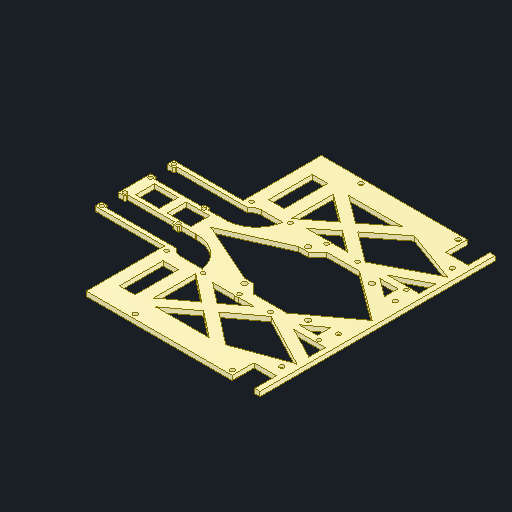
# Autodesk Inventor part: base
Saved by Autodesk Inventor 2023 (Build 270158000, 158)
## iProperties
Created: 2024-05-25
Part Number: base
Material: Nylon 6
Document SubType Name: Modeling
Designer: szymo
Density: 1.12 g/cm^3
Appearance: Nylon 6
Mass: 52.6414 g
Surface Area: 374.205 cm^2
Volume: 47.0013 cm^3
Author: szymo
Autodesk Inventor part; units mm, degrees
ref_plane "YZ Plane" through (0, 0, 0) normal (1, 0, 0) x (0, 1, 0)
ref_plane "XZ Plane" through (0, 0, 0) normal (0, 1, 0) x (-1, 0, 0)
ref_plane "XY Plane" through (0, 0, 0) normal (0, 0, 1) x (1, 0, 0)
sketch "Sketch1" plane through (0, 0, 0) normal (0, 1, 0) x (-1, 0, 0)
  line L0 (99, 89) -> (-99, 89)
  line L1 (-99, 89) -> (-99, -89)
  line L2 (-99, -89) -> (99, -89)
  line L3 (99, -89) -> (99, 89)
  line L4 (99, 89) -> (-99, -89) construction
  line L5 (-99, 89) -> (99, -89) construction
  line L6 (-85, 89) -> (-85, -89)
  line L7 (-64, 89) -> (-64, 72.5)
  line L8 (-64, 72.5) -> (-81, 72.5)
  line L9 (-81, -72.5) -> (-64, -72.5)
  line L10 (-64, -72.5) -> (-64, -89)
  line L11 (-81, -89) -> (-81, 89)
  point P0 (0, 0)
  dimension "d0" = 198
  dimension "d1" = 178
  dimension "d2" = 14
  dimension "d3" = 16.5
  dimension "d4" = 16.5
  dimension "d9" = 4
  dimension "d10" = 17
  dimension "d11" = 17
  constraints: 24 end point, 8 point on line, 6 perpendicular, 2 horizontal, 2 midpoint, 2 parallel, 1 vertical
  measures "d0" distance of L2.end L1.end
  measures "d1" distance of L1.end L0.end
  measures "d2" distance between parallel lines of L6 L1
  measures "d3" distance between parallel lines of L0 L8
  measures "d4" distance between parallel lines of L9 L2
  measures "d9" distance between parallel lines of L11 L6
  measures "d10" distance between parallel lines of L10 L11
  measures "d11" distance between parallel lines of L11 L7
extrude "Extrusion1" add sketch "Sketch1" along normal blind 3.5 contours L3 L2 L10 L9 L11 L8 L7 L0 | L11 L2 L6 L0
sketch "Sketch2" plane through (0, 0, 0) normal (0, -1, 0) x (1, 0, 0)
  circle A0 centre (77, -64.5) radius 1.2295
  circle A1 centre (77, -21.5) radius 1.2295
  circle A2 centre (77, 21.5) radius 1.2295
  circle A3 centre (77, 64.5) radius 1.2295
  line L0 (79, 89) -> (79, 88)
  line L1 (-46.5, 89) -> (79, 89)
  line L2 (-46.5, 89) -> (-46.5, 73)
  line L3 (-39.246, 73) -> (-46.5, 73)
  spline S0 degree 3 poles (-38.725, 73.0306) (-38.9029, 73.01) (-39.0786, 73) (-39.246, 73) knots 0 0 0 0 1 1 1 1
  line L4 (-38.725, 88) -> (-38.725, 73.0306)
  line L5 (-24.275, 73.0306) -> (-24.275, 88)
  line L6 (-16.5, 73) -> (-23.754, 73)
  arc A4 (-9.5, 82) -> (-16.5, 73) centre (-6.5148, 72.456) ccw
  arc A5 (-1.5, 86) -> (-9.5, 82) centre (-1.5, 76) ccw
  circle A6 centre (70, 79.5) radius 1.75
  circle A7 centre (-13, 85.5) radius 2.3
  circle A8 centre (60.5017, 85.4375) radius 2.3
  circle A9 centre (70, -82.5) radius 1.75
  arc A10 (58.4256, -82) -> (56.6186, -83.1429) centre (58.4256, -84) ccw
  arc A11 (52.101, -86) -> (56.6186, -83.1429) centre (52.101, -81) ccw
  arc A12 (-9.5, -82) -> (-1.5, -86) centre (-1.5, -76) ccw
  arc A13 (-16.5, -73) -> (-9.5, -82) centre (-6.5148, -72.456) ccw
  line L7 (-16.5, -73) -> (-23.754, -73)
  spline S1 degree 3 poles (-23.754, -73) (-23.9214, -73) (-24.0971, -73.01) (-24.275, -73.0306) knots 0 0 0 0 1 1 1 1
  line L8 (-24.275, -73.0306) -> (-24.275, -88)
  line L9 (-24.275, -88) -> (-38.725, -88)
  line L10 (-38.725, -88) -> (-38.725, -73.0306)
  spline S2 degree 3 poles (-38.725, -73.0306) (-38.9029, -73.01) (-39.0786, -73) (-39.246, -73) knots 0 0 0 0 1 1 1 1
  line L11 (-39.246, -73) -> (-46.5, -73)
  line L12 (-46.5, -89) -> (-46.5, -73)
  line L13 (-46.5, -89) -> (79, -89)
  line L14 (79, -89) -> (79, -88)
  arc A14 (68.9282, -76) -> (66.9487, -77.7143) centre (68.9282, -78) ccw
  arc A15 (62, -82) -> (66.9487, -77.7143) centre (62, -77) ccw
  line L15 (62, -82) -> (58.4256, -82)
  circle A16 centre (-13, -85.5) radius 2.3
  circle A17 centre (60.5017, -85.4375) radius 2.3
  line L16 (73, 83) -> (73, 78)
  line L17 (52.101, 86) -> (-1.5, 86)
  arc A18 (71, 76) -> (73, 78) centre (71, 78) ccw
  arc A19 (78, 88) -> (73, 83) centre (78, 83) ccw
  line L18 (79, 88) -> (78, 88)
  line L19 (-24.275, 88) -> (-38.725, 88)
  spline S3 degree 3 poles (-23.754, 73) (-23.9214, 73) (-24.0971, 73.01) (-24.275, 73.0306) knots 0 0 0 0 1 1 1 1
  arc A20 (56.6186, 83.1429) -> (52.101, 86) centre (52.101, 81) ccw
  arc A21 (56.6186, 83.1429) -> (58.4256, 82) centre (58.4256, 84) ccw
  line L20 (62, 82) -> (58.4256, 82)
  arc A22 (66.9487, 77.7143) -> (62, 82) centre (62, 77) ccw
  arc A23 (66.9487, 77.7143) -> (68.9282, 76) centre (68.9282, 78) ccw
  line L21 (71, 76) -> (68.9282, 76)
  arc A24 (73, -78) -> (71, -76) centre (71, -78) ccw
  line L22 (71, -76) -> (68.9282, -76)
  line L23 (52.101, -86) -> (-1.5, -86)
  line L24 (79, -88) -> (78, -88)
  arc A25 (73, -83) -> (78, -88) centre (78, -83) ccw
  line L25 (73, -83) -> (73, -78)
  point P0 (0, 0)
  point P1 (-13, -85.5)
  point P2 (-13, 85.5)
  constraints: 6 coincident
hole "m3" at (-13, 0, -85.5) at (60.5017, 0, -85.4375) at (-13, 0, 85.5) at (60.5017, 0, 85.4375) at (77, 0, 64.5) at (77, 0, 21.5) at (77, 0, -21.5) at (77, 0, -64.5) direction (0, 1, 0) diameter 3.6 end through all countersink diameter 6.7 countersink angle 90 clearance for "Countersunk Flat Head Screw ISO 2009/7046" size "M3" standard "ISO"
sketch "Sketch3" plane through (0, 0, 0) normal (0, -1, 0) x (1, 0, 0)
  circle A0 centre (-96.5, -27.3) radius 1.75
  circle A1 centre (-96.5, -9.7) radius 1.75
  circle A2 centre (-96.5, 9.7) radius 1.75
  circle A3 centre (-96.5, 27.3) radius 1.75
  circle A4 centre (-56, 9.7) radius 1.75
  circle A5 centre (-56, -9.7) radius 1.75
  circle A6 centre (-42.5596, -32.1689) radius 1.5
  circle A7 centre (-42.5596, 32.1689) radius 1.75
  circle A8 centre (-13.9698, 33) radius 1.75
  circle A9 centre (13.5198, 33) radius 1.75
  circle A10 centre (37.0073, 33) radius 1.75
  circle A11 centre (73.7355, 33) radius 1.75
  circle A12 centre (73.7355, -33) radius 1.75
  circle A13 centre (37.0073, -33) radius 1.75
  circle A14 centre (-96.5, -27.3) radius 1.75
  circle A15 centre (73.7355, -33) radius 1.75
  circle A16 centre (13.5198, -33) radius 1.75
  circle A17 centre (-42.5596, -32.1689) radius 1.75
  circle A18 centre (-13.9698, -33) radius 1.75
  arc A19 (-94, -25.8) -> (-95, -24.8) centre (-95, -25.8) ccw
  line L0 (-95, -24.8) -> (-99, -24.8)
  line L1 (-99, -29.8) -> (-99, -24.8)
  line L2 (-48.6566, -29.8) -> (-99, -29.8)
  arc A20 (-47.7313, -30.4207) -> (-48.6566, -29.8) centre (-48.6566, -30.8) ccw
  arc A21 (-46.5, -35.5) -> (-47.7313, -30.4207) centre (-63.78, -37) ccw
  line L3 (79, -35.5) -> (-46.5, -35.5)
  line L4 (79, -35.5) -> (79, -30.5)
  line L5 (79, -30.5) -> (-33.3917, -30.5)
  arc A22 (-40.5373, -26.8) -> (-33.3917, -30.5) centre (-33.3917, -21.75) ccw
  line L6 (-40.5373, -26.8) -> (-41.9987, -26.8)
  spline S0 degree 3 poles (-46.8237, -26.8) (-46.5789, -26.8) (-46.2862, -26.7761) (-45.5332, -26.6913) (-44.9243, -26.6) (-44.4112, -26.6) (-43.8981, -26.6) (-43.2892, -26.6913) (-42.5362, -26.7761) (-42.2435, -26.8) (-41.9987, -26.8) knots 0 0 0 0 0.161475 0.161475 0.5 0.5 0.5 0.838525 0.838525 1 1 1 1
  line L7 (-46.8237, -26.8) -> (-94, -26.8)
  line L8 (-94, -26.8) -> (-94, -25.8)
  line L9 (28.681, 30.5) -> (45.3337, 30.5)
  circle A23 centre (37.0073, 33) radius 1.75
  circle A24 centre (-96.5, 27.3) radius 1.75
  circle A25 centre (73.7355, 33) radius 1.75
  circle A26 centre (13.5198, 33) radius 1.75
  circle A27 centre (-42.5596, 32.1689) radius 1.75
  circle A28 centre (-13.9698, 33) radius 1.75
  arc A29 (-95, 24.8) -> (-94, 25.8) centre (-95, 25.8) ccw
  line L10 (-94, 26.8) -> (-94, 25.8)
  line L11 (-46.8237, 26.8) -> (-94, 26.8)
  spline S1 degree 3 poles (-46.8237, 26.8) (-46.5789, 26.8) (-46.2862, 26.7761) (-45.5332, 26.6913) (-44.9243, 26.6) (-44.4112, 26.6) (-43.8981, 26.6) (-43.2892, 26.6913) (-42.5362, 26.7761) (-42.2435, 26.8) (-41.9987, 26.8) knots 0 0 0 0 0.161475 0.161475 0.5 0.5 0.5 0.838525 0.838525 1 1 1 1
  line L12 (-40.5373, 26.8) -> (-41.9987, 26.8)
  arc A30 (-33.3917, 30.5) -> (-40.5373, 26.8) centre (-33.3917, 21.75) ccw
  line L13 (79, 30.5) -> (-33.3917, 30.5)
  line L14 (79, 35.5) -> (79, 30.5)
  line L15 (79, 35.5) -> (-46.5, 35.5)
  arc A31 (-47.7313, 30.4207) -> (-46.5, 35.5) centre (-63.78, 37) ccw
  arc A32 (-48.6566, 29.8) -> (-47.7313, 30.4207) centre (-48.6566, 30.8) ccw
  line L16 (-48.6566, 29.8) -> (-99, 29.8)
  line L17 (-99, 29.8) -> (-99, 24.8)
  line L18 (-95, 24.8) -> (-99, 24.8)
  point P0 (0, 0)
  constraints: 16 coincident
hole "m2.5" at (73.7355, 0, -33) at (37.0073, 0, -33) at (13.5198, 0, -33) at (-13.9698, 0, -33) at (-42.5596, 0, -32.1689) at (73.7355, 0, 33) at (37.0073, 0, 33) at (13.5198, 0, 33) at (-13.9698, 0, 33) at (-42.5596, 0, 32.1689) at (-56, 0, 9.7) at (-56, 0, -9.7) at (-96.5, 0, -9.7) at (-96.5, 0, 9.7) at (-96.5, 0, 27.3) at (-96.5, 0, -27.3) direction (0, 1, 0) diameter 3.1 end through all countersink diameter 5.8 countersink angle 90 clearance for "Countersunk Flat Head Screw ISO 2009/7046" size "M2.5" standard "ISO"
sketch "Sketch6" plane through (0, 0, 0) normal (0, -1, 0) x (1, 0, 0)
  line L0 (60, 27.5) -> (5, 27.5) projected
  line L1 (5, 27.5) -> (5, -27.5) projected
  line L2 (5, -27.5) -> (60, -27.5) projected
  line L3 (60, -27.5) -> (60, 27.5) projected
  circle A0 centre (48.73, 26.5) radius 0.325 projected
  circle A1 centre (45, 26.5) radius 0.325 projected
  circle A2 centre (46.27, 26.5) radius 0.325 projected
  circle A3 centre (52.54, 26.5) radius 0.325 projected
  circle A4 centre (56.6, 24.1) radius 1.6 projected
  circle A5 centre (50, 26.5) radius 0.325 projected
  circle A6 centre (51.27, 26.5) radius 0.325 projected
  circle A7 centre (42.46, 26.5) radius 0.325 projected
  circle A8 centre (43.73, 26.5) radius 0.325 projected
  circle A9 centre (8.4, 24.1) radius 1.6 projected
  circle A10 centre (7, 15) radius 0.35 projected
  circle A11 centre (9.5, 15) radius 0.35 projected
  circle A12 centre (9.5, 7.75) radius 0.35 projected
  circle A13 centre (7, 7.75) radius 0.35 projected
  circle A14 centre (9.5, 0.5) radius 0.35 projected
  circle A15 centre (56.6, -24.1) radius 1.6 projected
  circle A16 centre (51.27, -26.5) radius 0.325 projected
  circle A17 centre (52.54, -26.5) radius 0.325 projected
  circle A18 centre (48.73, -26.5) radius 0.325 projected
  circle A19 centre (50, -26.5) radius 0.325 projected
  circle A20 centre (45, -26.5) radius 0.325 projected
  circle A21 centre (46.27, -26.5) radius 0.325 projected
  circle A22 centre (9.5, -6.75) radius 0.35 projected
  circle A23 centre (9.5, -14) radius 0.35 projected
  circle A24 centre (7, 0.5) radius 0.35 projected
  circle A25 centre (7, -6.75) radius 0.35 projected
  circle A26 centre (42.46, -26.5) radius 0.325 projected
  circle A27 centre (43.73, -26.5) radius 0.325 projected
  circle A28 centre (7, -14) radius 0.35 projected
  circle A29 centre (8.4, -24.1) radius 1.6 projected
  point P0 (0, 0)
  constraints: 4 coincident
hole "insert_stack" at (8.4, 0, -24.1) at (8.4, 0, 24.1) at (56.6, 0, 24.1) at (56.6, 0, -24.1) direction (0, 1, 0) diameter 4 depth 4.5 counterbore diameter 4.6 counterbore depth 1
sketch "Sketch5" plane through (0, 0, 0) normal (0, 1, 0) x (1, 0, 0)
  line L0 (-36.8852, -40.5) -> (-31.5, -40.5)
  line L1 (-31.5, -40.5) -> (-26.1148, -40.5)
  line L2 (-26.1148, -40.5) -> (-26.1148, -68.2)
  line L3 (-26.1148, -68.2) -> (-36.8852, -68.2)
  line L4 (-36.8852, -68.2) -> (-36.8852, -40.5)
  line L5 (-26.1148, 40.5) -> (-31.5, 40.5)
  line L6 (-31.5, 40.5) -> (-36.8852, 40.5)
  line L7 (-36.8852, 40.5) -> (-36.8852, 68.2)
  line L8 (-36.8852, 68.2) -> (-26.1148, 68.2)
  line L9 (-26.1148, 68.2) -> (-26.1148, 40.5)
  arc A0 (-99, -28.7697) -> (-99, -25.8303) centre (-96.5, -27.3) ccw
  line L10 (-99, -11.1697) -> (-99, -25.8303)
  arc A1 (-99, -11.1697) -> (-99, -8.2303) centre (-96.5, -9.7) ccw
  line L11 (-99, 8.2303) -> (-99, -8.2303)
  arc A2 (-99, 8.2303) -> (-99, 11.1697) centre (-96.5, 9.7) ccw
  line L12 (-99, 25.8303) -> (-99, 11.1697)
  arc A3 (-99, 25.8303) -> (-99, 28.7697) centre (-96.5, 27.3) ccw
  line L13 (-99, 89) -> (-99, 28.7697)
  line L14 (64, 89) -> (-99, 89)
  line L15 (64, 72.5) -> (64, 89)
  line L16 (81, 72.5) -> (64, 72.5)
  line L17 (81, 89) -> (81, 72.5)
  line L18 (85, 89) -> (81, 89)
  line L19 (85, -89) -> (85, 89)
  line L20 (81, -89) -> (85, -89)
  line L21 (81, -72.5) -> (81, -89)
  line L22 (64, -72.5) -> (81, -72.5)
  line L23 (64, -89) -> (64, -72.5)
  line L24 (-99, -89) -> (64, -89)
  line L25 (-99, -28.7697) -> (-99, -89)
  circle A4 centre (77, 64.5) radius 3.35
  circle A5 centre (77, -21.5) radius 3.35
  circle A6 centre (60.5017, -85.4375) radius 3.35
  circle A7 centre (60.5017, 85.4375) radius 3.35
  circle A8 centre (-13, 85.5) radius 3.35
  circle A9 centre (-13, -85.5) radius 3.35
  circle A10 centre (77, -64.5) radius 3.35
  circle A11 centre (77, 21.5) radius 3.35
  circle A12 centre (-56, 9.7) radius 2.9
  circle A13 centre (-42.5596, -32.1689) radius 2.9
  circle A14 centre (13.5198, -33) radius 2.9
  circle A15 centre (73.7355, -33) radius 2.9
  circle A16 centre (-13.9698, 33) radius 2.9
  circle A17 centre (37.0073, 33) radius 2.9
  circle A18 centre (73.7355, 33) radius 2.9
  circle A19 centre (13.5198, 33) radius 2.9
  circle A20 centre (-42.5596, 32.1689) radius 2.9
  circle A21 centre (37.0073, -33) radius 2.9
  circle A22 centre (-13.9698, -33) radius 2.9
  circle A23 centre (-56, -9.7) radius 2.9
  arc A24 (56.6186, 83.1429) -> (58.4256, 82) centre (58.4256, 84) ccw
  arc A25 (56.6186, 83.1429) -> (52.101, 86) centre (52.101, 81) ccw
  line L26 (52.101, 86) -> (-1.5, 86)
  arc A26 (-1.5, 86) -> (-9.5, 82) centre (-1.5, 76) ccw
  arc A27 (-9.5, 82) -> (-16.5, 73) centre (-6.5148, 72.456) ccw
  line L27 (-16.5, 73) -> (-23.754, 73)
  spline S0 degree 3 poles (-23.754, 73) (-23.9214, 73) (-24.0971, 73.01) (-24.275, 73.0306) knots 0 0 0 0 1 1 1 1
  line L28 (-24.275, 73.0306) -> (-24.275, 88)
  line L29 (-24.275, 88) -> (-38.725, 88)
  line L30 (-38.725, 88) -> (-38.725, 73.0306)
  spline S1 degree 3 poles (-38.725, 73.0306) (-38.9029, 73.01) (-39.0786, 73) (-39.246, 73) knots 0 0 0 0 1 1 1 1
  line L31 (-39.246, 73) -> (-46.5, 73)
  line L32 (-46.5, 89) -> (-46.5, 73)
  line L33 (-46.5, 89) -> (79, 89)
  line L34 (79, 89) -> (79, 86)
  arc A28 (79, 86) -> (74.3229, 81.0104) centre (79.3229, 81.0104) ccw
  line L35 (74.3229, 81.0104) -> (74.3229, 78)
  arc A29 (72.3229, 76) -> (74.3229, 78) centre (72.3229, 78) ccw
  line L36 (72.3229, 76) -> (68.9282, 76)
  arc A30 (66.9487, 77.7143) -> (68.9282, 76) centre (68.9282, 78) ccw
  arc A31 (66.9487, 77.7143) -> (62, 82) centre (62, 77) ccw
  line L37 (62, 82) -> (58.4256, 82)
  arc A32 (-95, 24.8) -> (-94, 25.8) centre (-95, 25.8) ccw
  line L38 (-95, 24.8) -> (-99, 24.8)
  line L39 (-99, 29.8) -> (-99, 24.8)
  line L40 (-48.6566, 29.8) -> (-99, 29.8)
  arc A33 (-48.6566, 29.8) -> (-47.7313, 30.4207) centre (-48.6566, 30.8) ccw
  arc A34 (-47.7313, 30.4207) -> (-46.5, 35.5) centre (-63.78, 37) ccw
  line L41 (79, 35.5) -> (-46.5, 35.5)
  line L42 (79, 35.5) -> (79, 30.5)
  line L43 (79, 30.5) -> (-33.3917, 30.5)
  arc A35 (-33.3917, 30.5) -> (-40.5373, 26.8) centre (-33.3917, 21.75) ccw
  line L44 (-40.5373, 26.8) -> (-41.9987, 26.8)
  spline S2 degree 3 poles (-46.8237, 26.8) (-46.5789, 26.8) (-46.2862, 26.7761) (-45.5332, 26.6913) (-44.9243, 26.6) (-44.4112, 26.6) (-43.8981, 26.6) (-43.2892, 26.6913) (-42.5362, 26.7761) (-42.2435, 26.8) (-41.9987, 26.8) knots 0 0 0 0 0.161475 0.161475 0.5 0.5 0.5 0.838525 0.838525 1 1 1 1
  line L45 (-46.8237, 26.8) -> (-94, 26.8)
  line L46 (-94, 26.8) -> (-94, 25.8)
  arc A36 (-57.5, 12.2) -> (-58.5, 11.2) centre (-57.5, 11.2) ccw
  line L47 (-57.5, 12.2) -> (-54.5, 12.2)
  arc A37 (-53.5, 11.2) -> (-54.5, 12.2) centre (-54.5, 11.2) ccw
  line L48 (-53.5, 11.2) -> (-53.5, 10.2)
  line L49 (-53.5, 10.2) -> (-46.8237, 10.2)
  spline S3 degree 3 poles (-41.9987, 10.2) (-42.2435, 10.2) (-42.5362, 10.2239) (-43.2892, 10.3087) (-43.8981, 10.4) (-44.4112, 10.4) (-44.9243, 10.4) (-45.5332, 10.3087) (-46.2862, 10.2239) (-46.5789, 10.2) (-46.8237, 10.2) knots 0 0 0 0 0.161475 0.161475 0.5 0.5 0.5 0.838525 0.838525 1 1 1 1
  line L50 (-41.9987, 10.2) -> (-41.148, 10.2)
  line L51 (-41.148, 10.2) -> (-41.148, 7.2)
  line L52 (-41.148, 7.2) -> (-99, 7.2)
  line L53 (-99, 7.2) -> (-99, 12.2)
  line L54 (-99, 12.2) -> (-95, 12.2)
  arc A38 (-94, 11.2) -> (-95, 12.2) centre (-95, 11.2) ccw
  line L55 (-94, 10.2) -> (-94, 11.2)
  line L56 (-94, 10.2) -> (-58.5, 10.2)
  line L57 (-58.5, 10.2) -> (-58.5, 11.2)
  arc A39 (-58.5, -11.2) -> (-57.5, -12.2) centre (-57.5, -11.2) ccw
  line L58 (-58.5, -10.2) -> (-58.5, -11.2)
  line L59 (-94, -10.2) -> (-58.5, -10.2)
  line L60 (-94, -10.2) -> (-94, -11.2)
  arc A40 (-95, -12.2) -> (-94, -11.2) centre (-95, -11.2) ccw
  line L61 (-99, -12.2) -> (-95, -12.2)
  line L62 (-99, -7.2) -> (-99, -12.2)
  line L63 (-41.148, -7.2) -> (-99, -7.2)
  line L64 (-41.148, -10.2) -> (-41.148, -7.2)
  line L65 (-41.9987, -10.2) -> (-41.148, -10.2)
  spline S4 degree 3 poles (-41.9987, -10.2) (-42.2435, -10.2) (-42.5362, -10.2239) (-43.2892, -10.3087) (-43.8981, -10.4) (-44.4112, -10.4) (-44.9243, -10.4) (-45.5332, -10.3087) (-46.2862, -10.2239) (-46.5789, -10.2) (-46.8237, -10.2) knots 0 0 0 0 0.161475 0.161475 0.5 0.5 0.5 0.838525 0.838525 1 1 1 1
  line L66 (-53.5, -10.2) -> (-46.8237, -10.2)
  line L67 (-53.5, -11.2) -> (-53.5, -10.2)
  arc A41 (-54.5, -12.2) -> (-53.5, -11.2) centre (-54.5, -11.2) ccw
  line L68 (-57.5, -12.2) -> (-54.5, -12.2)
  arc A42 (-94, -25.8) -> (-95, -24.8) centre (-95, -25.8) ccw
  line L69 (-94, -26.8) -> (-94, -25.8)
  line L70 (-46.8237, -26.8) -> (-94, -26.8)
  spline S5 degree 3 poles (-46.8237, -26.8) (-46.5789, -26.8) (-46.2862, -26.7761) (-45.5332, -26.6913) (-44.9243, -26.6) (-44.4112, -26.6) (-43.8981, -26.6) (-43.2892, -26.6913) (-42.5362, -26.7761) (-42.2435, -26.8) (-41.9987, -26.8) knots 0 0 0 0 0.161475 0.161475 0.5 0.5 0.5 0.838525 0.838525 1 1 1 1
  line L71 (-40.5373, -26.8) -> (-41.9987, -26.8)
  arc A43 (-40.5373, -26.8) -> (-33.3917, -30.5) centre (-33.3917, -21.75) ccw
  line L72 (79, -30.5) -> (-33.3917, -30.5)
  line L73 (79, -35.5) -> (79, -30.5)
  line L74 (79, -35.5) -> (-46.5, -35.5)
  arc A44 (-46.5, -35.5) -> (-47.7313, -30.4207) centre (-63.78, -37) ccw
  arc A45 (-47.7313, -30.4207) -> (-48.6566, -29.8) centre (-48.6566, -30.8) ccw
  line L75 (-48.6566, -29.8) -> (-99, -29.8)
  line L76 (-99, -29.8) -> (-99, -24.8)
  line L77 (-95, -24.8) -> (-99, -24.8)
  arc A46 (58.4256, -82) -> (56.6186, -83.1429) centre (58.4256, -84) ccw
  line L78 (62, -82) -> (58.4256, -82)
  arc A47 (62, -82) -> (66.9487, -77.7143) centre (62, -77) ccw
  arc A48 (68.9282, -76) -> (66.9487, -77.7143) centre (68.9282, -78) ccw
  line L79 (72.3229, -76) -> (68.9282, -76)
  arc A49 (74.3229, -78) -> (72.3229, -76) centre (72.3229, -78) ccw
  line L80 (74.3229, -81.0104) -> (74.3229, -78)
  arc A50 (74.3229, -81.0104) -> (79, -86) centre (79.3229, -81.0104) ccw
  line L81 (79, -89) -> (79, -86)
  line L82 (-46.5, -89) -> (79, -89)
  line L83 (-46.5, -89) -> (-46.5, -73)
  line L84 (-39.246, -73) -> (-46.5, -73)
  spline S6 degree 3 poles (-38.725, -73.0306) (-38.9029, -73.01) (-39.0786, -73) (-39.246, -73) knots 0 0 0 0 1 1 1 1
  line L85 (-38.725, -88) -> (-38.725, -73.0306)
  line L86 (-24.275, -88) -> (-38.725, -88)
  line L87 (-24.275, -73.0306) -> (-24.275, -88)
  spline S7 degree 3 poles (-23.754, -73) (-23.9214, -73) (-24.0971, -73.01) (-24.275, -73.0306) knots 0 0 0 0 1 1 1 1
  line L88 (-16.5, -73) -> (-23.754, -73)
  arc A51 (-16.5, -73) -> (-9.5, -82) centre (-6.5148, -72.456) ccw
  arc A52 (-9.5, -82) -> (-1.5, -86) centre (-1.5, -76) ccw
  line L89 (52.101, -86) -> (-1.5, -86)
  arc A53 (52.101, -86) -> (56.6186, -83.1429) centre (52.101, -81) ccw
  line L90 (85, 89) -> (99, 89)
  line L91 (99, 89) -> (99, -89)
  line L92 (85, -89) -> (99, -89)
  line L93 (85, 89) -> (85, -89)
  line L94 (70, 72) -> (79, 72)
  arc A54 (79, 72) -> (81, 74) centre (79, 74) ccw
  line L95 (81, 74) -> (81, 89)
  line L96 (81, 89) -> (85, 89)
  line L97 (85, 89) -> (85, -89)
  line L98 (81, -89) -> (85, -89)
  line L99 (81, -89) -> (81, -74)
  arc A55 (81, -74) -> (79, -72) centre (79, -74) ccw
  line L100 (79, -72) -> (70, -72)
  line L101 (70, -57) -> (70, -72)
  line L102 (70, -57) -> (79, -57)
  arc A56 (79, -57) -> (81, -55) centre (79, -55) ccw
  line L103 (81, -55) -> (81, -31)
  arc A57 (81, -31) -> (79, -29) centre (79, -31) ccw
  line L104 (79, -29) -> (70, -29)
  line L105 (70, -14) -> (70, -29)
  line L106 (70, -14) -> (79, -14)
  arc A58 (79, -14) -> (81, -12) centre (79, -12) ccw
  line L107 (81, -12) -> (81, 12)
  arc A59 (81, 12) -> (79, 14) centre (79, 12) ccw
  line L108 (79, 14) -> (70, 14)
  line L109 (70, 29) -> (70, 14)
  line L110 (70, 29) -> (79, 29)
  arc A60 (79, 29) -> (81, 31) centre (79, 31) ccw
  line L111 (81, 31) -> (81, 55)
  arc A61 (81, 55) -> (79, 57) centre (79, 55) ccw
  line L112 (79, 57) -> (70, 57)
  line L113 (70, 72) -> (70, 57)
  line L114 (60, -27.5) -> (5, -27.5)
  line L115 (5, -27.5) -> (5, 27.5)
  line L116 (5, 27.5) -> (60, 27.5)
  line L117 (60, 27.5) -> (60, -27.5)
  circle A62 centre (56.6, -24.1) radius 1.6
  circle A63 centre (8.4, -24.1) radius 1.6
  circle A64 centre (56.6, 24.1) radius 1.6
  circle A65 centre (8.4, 24.1) radius 1.6
  line L118 (-37.3852, 68.7) -> (-37.3852, 40)
  line L119 (-37.3852, 40) -> (-31.5, 40)
  line L120 (-31.5, 40) -> (-25.6148, 40)
  line L121 (-25.6148, 40) -> (-25.6148, 68.7)
  line L122 (-25.6148, 68.7) -> (-37.3852, 68.7)
  line L123 (-37.3852, -40) -> (-31.5, -40)
  line L124 (-31.5, -40) -> (-25.6148, -40)
  line L125 (-25.6148, -40) -> (-25.6148, -68.7)
  line L126 (-25.6148, -68.7) -> (-37.3852, -68.7)
  line L127 (-37.3852, -68.7) -> (-37.3852, -40)
  line L128 (81, 55) -> (81, 57)
  line L129 (81, 57) -> (79, 57)
  line L130 (-46.5, -73) -> (64, -73)
  line L131 (-46.5, 73) -> (64, 73)
  line L132 (81, 57) -> (37.0404, 73)
  line L133 (79, -57) -> (81, -57)
  line L134 (81, -57) -> (81, -55)
  line L135 (81, -57) -> (37.0404, -73)
  line L136 (-46.5, 73) -> (-46.5, 35.5)
  line L137 (-37.3852, 73) -> (-37.3852, 68.7)
  line L138 (-37.3852, 40) -> (-37.3852, 35.5)
  line L139 (-25.6148, 40) -> (-25.6148, 35.5)
  line L140 (-25.6148, 68.7) -> (-25.6148, 73)
  line L141 (-16.5, 73) -> (-16.5, 35.5)
  line L142 (-46.5, -35.5) -> (-46.5, -73)
  line L143 (-37.3852, -35.5) -> (-37.3852, -40)
  line L144 (-37.3852, -68.7) -> (-37.3852, -73)
  line L145 (-25.6148, -68.7) -> (-25.6148, -73)
  line L146 (-25.6148, -40) -> (-25.6148, -35.5)
  line L147 (-16.5, -73) -> (-16.5, -35.5)
  line L148 (79, 35.5) -> (81, 35.5)
  line L149 (79, 30.5) -> (80.9365, 30.5)
  line L150 (79, -35.5) -> (81, -35.5)
  line L151 (79, -30.5) -> (80.9365, -30.5)
  line L152 (53.1, 27.6) -> (60.1, 27.6)
  line L153 (60.1, 27.6) -> (60.1, 20.6)
  line L154 (60.1, 20.6) -> (53.1, 20.6)
  line L155 (53.1, 20.6) -> (53.1, 27.6)
  line L156 (53.1, 27.6) -> (60.1, 20.6) construction
  line L157 (60.1, 27.6) -> (53.1, 20.6) construction
  line L158 (53.1, -20.6) -> (60.1, -20.6)
  line L159 (60.1, -20.6) -> (60.1, -27.6)
  line L160 (60.1, -27.6) -> (53.1, -27.6)
  line L161 (53.1, -27.6) -> (53.1, -20.6)
  line L162 (53.1, -20.6) -> (60.1, -27.6) construction
  line L163 (60.1, -20.6) -> (53.1, -27.6) construction
  line L164 (4.9, 27.6) -> (11.9, 27.6)
  line L165 (11.9, 27.6) -> (11.9, 20.6)
  line L166 (11.9, 20.6) -> (4.9, 20.6)
  line L167 (4.9, 20.6) -> (4.9, 27.6)
  line L168 (4.9, 27.6) -> (11.9, 20.6) construction
  line L169 (11.9, 27.6) -> (4.9, 20.6) construction
  line L170 (4.9, -27.6) -> (11.9, -27.6)
  line L171 (11.9, -27.6) -> (11.9, -20.6)
  line L172 (11.9, -20.6) -> (4.9, -20.6)
  line L173 (4.9, -20.6) -> (4.9, -27.6)
  line L174 (4.9, -27.6) -> (11.9, -20.6) construction
  line L175 (11.9, -27.6) -> (4.9, -20.6) construction
  line L176 (81, 57) -> (39.6917, 35.5)
  line L177 (81, -57) -> (39.6917, -35.5)
  line L178 (81, 0) -> (39.6917, 30.5)
  line L179 (81, 0) -> (39.6917, -30.5)
  line L180 (39.6917, 35.5) -> (39.6917, 30.5)
  line L181 (39.6917, -30.5) -> (39.6917, -35.5)
  line L182 (11.9, 20.6) -> (21.8, 30.5)
  line L183 (11.9, -20.6) -> (21.8, -30.5)
  line L184 (4.9, 20.6) -> (-5, 30.5)
  line L185 (4.9, -20.6) -> (-5, -30.5)
  line L186 (37.0404, 73) -> (-13.9698, 33) construction
  line L187 (37.0404, -73) -> (-13.9698, -33) construction
  line L188 (-16.5, 73) -> (37.0073, 33) construction
  line L189 (-16.5, -73) -> (37.0073, -33) construction
  line L190 (-16.5, 68.0058) -> (26.9825, 35.5)
  line L191 (-9.8194, 73) -> (40.3437, 35.5)
  line L192 (-16.5, 36.0991) -> (30.558, 73)
  line L193 (43.5227, 73) -> (-4.2994, 35.5)
  line L194 (30.558, -73) -> (-16.5, -36.0991)
  line L195 (-16.5, -68.0058) -> (26.9825, -35.5)
  line L196 (40.3437, -35.5) -> (-9.8194, -73)
  line L197 (-4.2994, -35.5) -> (43.5227, -73)
  line L198 (-46.8237, 26.8) -> (-41.9987, 26.8)
  line L199 (-41.9987, 10.2) -> (-46.8237, 10.2)
  line L200 (-46.8237, -10.2) -> (-41.9987, -10.2)
  line L201 (-41.9987, -26.8) -> (-46.8237, -26.8)
  line L202 (-46.5, 35.5) -> (-46.5, 29.8)
  line L203 (-46.5, 29.8) -> (-48.6566, 29.8)
  line L204 (-48.6566, -29.8) -> (-46.5, -29.8)
  line L205 (-46.5, -29.8) -> (-46.5, -35.5)
  line L206 (-99, 7.2) -> (-91, 7.2)
  line L207 (-91, 7.2) -> (-91, -7.2)
  line L208 (-91, -7.2) -> (-99, -7.2)
  line L209 (-99, -7.2) -> (-99, 7.2)
  line L210 (-41.148, 7.2) -> (-49.148, 7.2)
  line L211 (-49.148, 7.2) -> (-49.148, -7.2)
  line L212 (-49.148, -7.2) -> (-41.148, -7.2)
  line L213 (-41.148, -7.2) -> (-41.148, 7.2)
  line L214 (-73.074, 7.2) -> (-67.074, 7.2)
  line L215 (-67.074, 7.2) -> (-67.074, -7.2)
  line L216 (-67.074, -7.2) -> (-73.074, -7.2)
  line L217 (-73.074, -7.2) -> (-73.074, 7.2)
  circle A66 centre (-41.148, 34.5207) radius 24.3207
  line L218 (-41.148, 34.5207) -> (-41.148, 10.2)
  line L219 (-41.148, 0) -> (4.9, 20.6)
  line L220 (-41.148, 0) -> (4.9, -20.6)
  circle A67 centre (-41.148, -34.5207) radius 24.3207
  line L221 (-41.148, -34.5207) -> (-41.148, -10.2)
  line L222 (57.0195, 35.5) -> (81, 47.9813)
  line L223 (57.0195, -35.5) -> (81, -47.9813)
  line L224 (56.1723, -30.5) -> (81, -12.1685)
  line L225 (81, 12.1685) -> (56.1723, 30.5)
  line L226 (70, -20.2903) -> (70, -30.5)
  line L227 (70, 20.2903) -> (70, 30.5)
  point P0 (0, 0)
  point P1 (10.8517, -57.5471)
  point P2 (4.3307, -52.4336)
  point P3 (10.9679, -47.4719)
  point P4 (14.9895, -35.5)
  point P5 (12.0501, -35.5)
  point P6 (80.2128, -56.5903)
  point P7 (40.0761, -35.7)
  point P8 (17.4889, -52.5854)
  point P9 (41.4677, -71.3886)
  point P10 (10.9679, 47.4719)
  point P11 (12.0501, 35.5)
  point P12 (14.9895, 35.5)
  point P13 (41.4677, 71.3886)
  point P14 (17.4889, 52.5854)
  point P15 (40.0761, 35.7)
  point P16 (80.2128, 56.5903)
  point P17 (10.8517, 57.5471)
  point P18 (4.3307, 52.4336)
  point P19 (-26.1148, -53.6387)
  point P20 (-25.6148, -53.2348)
  point P21 (-37.3852, -58.5485)
  point P22 (-36.8852, -58.4649)
  point P23 (-17.1619, -30.5)
  point P24 (-42.855, -10.26)
  point P25 (-53.1434, -10.2)
  point P26 (-53.5, -11.1697)
  point P27 (-54.5303, -12.2)
  point P28 (-57.4697, -12.2)
  point P29 (-58.5, -11.1697)
  point P30 (-58.8566, -10.2)
  point P31 (-93.6434, -10.2)
  point P32 (-94, -11.1697)
  point P33 (-95.0303, -12.2)
  point P34 (-97.9697, -12.2)
  point P35 (-97.9697, -24.8)
  point P36 (-95.0303, -24.8)
  point P37 (-94, -25.8303)
  point P38 (-93.6434, -26.8)
  point P39 (-95.0303, -29.8)
  point P40 (-97.9697, -29.8)
  point P41 (-95.0303, 24.8)
  point P42 (-97.9697, 24.8)
  point P43 (-97.9697, 12.2)
  point P44 (-95.0303, 12.2)
  point P45 (-94, 11.1697)
  point P46 (-93.6434, 10.2)
  point P47 (-58.8566, 10.2)
  point P48 (-58.5, 11.1697)
  point P49 (-57.4697, 12.2)
  point P50 (-54.5303, 12.2)
  point P51 (-53.5, 11.1697)
  point P52 (-53.1434, 10.2)
  point P53 (-42.855, 10.26)
  point P54 (-17.1619, 30.5)
  point P55 (-93.6434, 26.8)
  point P56 (-94, 25.8303)
  point P57 (-97.9697, 29.8)
  point P58 (-95.0303, 29.8)
  point P59 (-57.4697, -7.2)
  point P60 (-54.5303, -7.2)
  point P61 (-54.5303, 7.2)
  point P62 (-57.4697, 7.2)
  point P63 (18.8, -27.5)
  point P64 (43.7549, -27.5)
  point P65 (43.7549, 27.5)
  point P66 (18.8, 27.5)
  dimension "d47" = 0.5
  dimension "d48" = 0.5
  dimension "d49" = 20
  dimension "d50" = 20
  dimension "d51" = 7
  dimension "d52" = 7
  dimension "d53" = 7
  dimension "d54" = 7
  dimension "d55" = 7
  dimension "d56" = 7
  dimension "d57" = 7
  dimension "d58" = 7
  dimension "d59" = 27.496
  dimension "d60" = 27.496
  dimension "d61" = 45
  dimension "d62" = 45
  dimension "d63" = 45
  dimension "d64" = 45
  dimension "d65" = 4
  dimension "d66" = 4
  dimension "d67" = 4
  dimension "d68" = 4
  dimension "d69" = 4
  dimension "d70" = 4
  dimension "d71" = 4
  dimension "d73" = 4
  dimension "d74" = 8
  dimension "d75" = 8
  dimension "d76" = 6
  dimension "d77" = 17.926
  dimension "d78" = 17.926
  dimension "d81" = 8
  dimension "d84" = 8
  constraints: 238 end point, 48 point on line, 34 parallel, 17 horizontal, 14 vertical, 12 perpendicular, 10 midpoint, 5 tangent, 2 collinear, 2 point on circle, 54 other
  measures "d47" distance between parallel lines of L7 L118
  measures "d48" distance between parallel lines of L4 L127
  measures "d49" angle to the sketch x axis of L135
  measures "d50" angle of L131 L132
  measures "d51" distance of L153.end L154.end
  measures "d52" distance of L152.end L153.end
  measures "d53" distance of L159.end L160.end
  measures "d54" distance of L158.end L159.end
  measures "d55" distance of L165.end L166.end
  measures "d56" distance of L164.end L165.end
  measures "d57" distance of L172.end L171.end
  measures "d58" distance of L171.end L170.end
  measures "d59" angle to the sketch x axis of L176
  measures "d60" angle to the sketch x axis of L177
  measures "d61" angle of L43 L182
  measures "d62" angle of L72 L183
  measures "d63" angle of L72 L185
  measures "d64" angle of L43 L184
  measures "d65" distance between parallel lines of L188 L190
  measures "d66" distance between parallel lines of L188 L191
  measures "d67" distance between parallel lines of L186 L192
  measures "d68" distance between parallel lines of L186 L193
  measures "d69" distance between parallel lines of L187 L194
  measures "d70" distance between parallel lines of L189 L195
  measures "d71" distance between parallel lines of L189 L196
  measures "d73" distance between parallel lines of L197 L187
  measures "d74" distance of L207.end L208.end
  measures "d75" distance of L212.end L211.end
  measures "d76" distance of L215.end L216.end
  measures "d77" distance between parallel lines of L207 L217
  measures "d78" distance between parallel lines of L211 L215
  measures "d81" distance between parallel lines of L176 L222
  measures "d84" distance between parallel lines of L177 L223
extrude "zeberka" cut sketch "Sketch5" along normal blind 3.5 contours L4 A67 L127 L123 L124 L125 L2 L1 L0 | L0 L1 L2 A67 L4 | A67 L2 L3 L4 | L4 L3 L2 A67 L125 L126 L127 | L126 L145 L130 L144 | A67 L75 A45 A44 L142 | L142 L83 L24 L25 L75 A0 A67 | A44 A45 L204 L205 | A0 L75 | A67 S4 L221 L71 S5 L70 | L70 A0 L69 A42 L77 L10 L61 A1 A40 L60 L59 A23 L58 A39 L68 A41 L67 L66 S4 A67 | L70 L69 A0 | S5 L201 | A67 S4 | S4 L200 A67 | L194 L195 L147 | L72 A43 L71 L221 A67 | L196 L194 L130 | L77 A0 | A23 L67 L66 | L74 A14 L195 L197 | L196 L177 A56 L102 L101 L135 L197 | L63 A23 L215 L52 A12 L211 | L219 L166 L115 L172 L220 | A23 L68 | L63 A23 | L101 L102 L133 L135 | L61 A1 | L177 L133 A56 | L115 L166 L182 L116 L178 L117 L179 L114 L183 L172 | A12 L52 | L218 L44 A35 L43 A66 | A66 S3 L45 S2 L44 L218 | A23 L59 L58 | L74 A15 L150 L103 L223 | L60 L59 A1 | L63 L207 L52 L217 | L74 A15 | L56 A2 L55 A38 L54 L12 L38 A3 A32 L46 L45 A66 S3 L49 A12 L48 A37 L47 A36 L57 | A12 L57 L56 | L49 L48 A12 | S2 L198 | L41 L193 L190 A19 | L224 L105 L226 L72 | L56 L55 A2 | A12 L47 | A3 L46 L45 | A66 L136 A34 A33 L40 | L40 A3 L13 L14 L32 L136 A66 | L117 L178 L179 | A2 L54 | L40 A3 | A33 A34 L202 L203 | L141 L190 L192 | A66 L9 L8 L7 L118 L122 L121 | L121 L120 L119 L118 A66 L7 L6 L5 L9 | L43 L227 L109 L225 | L193 L132 L113 L112 A61 L176 L191 | A3 L38 | L122 L137 L131 L140 | A66 L7 L8 L9 | L9 L5 L6 L7 A66 | L191 L131 L192 | A61 L129 L176 | L132 L129 L112 L113 | L41 L222 L111 L148 A18 | A18 L41
body "Solid1"
